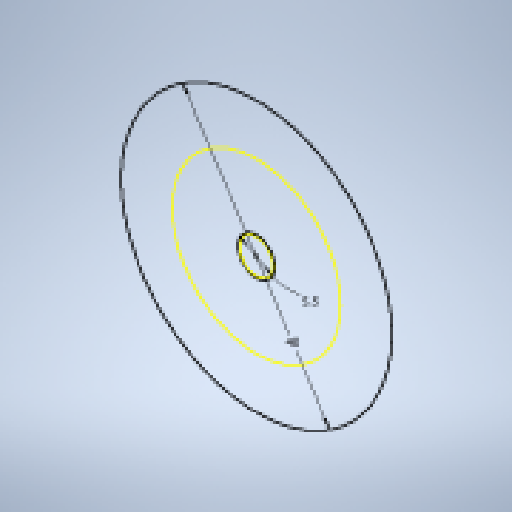
# Autodesk Inventor part: motorni_zobnik
Saved by Autodesk Inventor 2023 (Build 270158000, 158)
## iProperties
Created: 2022-09-15
Part Number: motorni_zobnik
Material: Generic
Document SubType Name: Modeling
Designer: simon
Density: 1 g/cm^3
Appearance: Default
Author: simon
Autodesk Inventor part; units mm, degrees
ref_plane "YZ Plane" through (0, 0, 0) normal (1, 0, 0) x (0, 1, 0)
ref_plane "XZ Plane" through (0, 0, 0) normal (0, 1, 0) x (-1, 0, 0)
ref_plane "XY Plane" through (0, 0, 0) normal (0, 0, 1) x (1, 0, 0)
sketch "Sketch1" plane through (0, 0, 0) normal (0, 0, 1) x (1, 0, 0)
  circle A0 centre (0, 0) radius 2.5 projected
  circle A1 centre (0, 0) radius 12.5 projected
  circle A2 centre (0, 0) radius 2.75
  circle A3 centre (0, 0) radius 20
  dimension "d0" = 5.5
  dimension "d1" = 40
  constraints: 2 centre point, 2 coincident
  measures "d0" diameter of A2
  measures "d1" diameter of A3
extrude "Extrusion1" add sketch "Sketch1" along normal blind 5 contours A1 | A3
body "Solid1"
